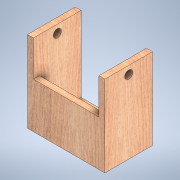
# Autodesk Inventor part: woodForkAssembly02
Saved by Autodesk Inventor 2022.2 (Build 262287000, 287)
## iProperties
Created: 2020-07-02
Part Number: woodForkAssembly02
Material: Wood (Birch)
Document SubType Name: Modeling
Designer: robst
Density: 0.55 g/cm^3
Appearance: Birch - Natural Polished
Mass: 1433.83 g
Surface Area: 3055.89 cm^2
Volume: 2606.97 cm^3
Author: robst
Autodesk Inventor part; units mm, degrees
ref_plane "YZ Plane" through (0, 0, 0) normal (1, 0, 0) x (0, 1, 0)
ref_plane "XZ Plane" through (0, 0, 0) normal (0, 1, 0) x (-1, 0, 0)
ref_plane "XY Plane" through (0, 0, 0) normal (0, 0, 1) x (1, 0, 0)
sketch "Sketch1" plane through (0, 0, 0) normal (0, 1, 0) x (-1, 0, 0)
  line L0 (123.825, 76.2) -> (-123.825, 76.2)
  line L1 (-123.825, 76.2) -> (-123.825, -76.2)
  line L2 (-123.825, -76.2) -> (123.825, -76.2)
  line L3 (123.825, -76.2) -> (123.825, 76.2)
  line L4 (123.825, 76.2) -> (-123.825, -76.2) construction
  line L5 (-123.825, 76.2) -> (123.825, -76.2) construction
  point P0 (0, 0)
  dimension "d0" = 247.65
  dimension "d1" = 152.4
  constraints: 12 end point, 2 midpoint, 2 parallel, 1 horizontal, 1 perpendicular
  measures "d0" distance of L0.start L0.end
  measures "d1" distance of L1.end L0.end
extrude "Extrusion1" add sketch "Sketch1" against normal blind 19.05
sketch "Sketch2" plane through (0, 0, 0) normal (0, 1, 0) x (1, 0, 0)
  line L0 (-123.825, -76.2) -> (-123.825, 76.2) projected
  line L1 (-123.825, 76.2) -> (-104.775, 76.2)
  line L2 (-104.775, 76.2) -> (-104.775, -76.2)
  line L3 (-104.775, -76.2) -> (-123.825, -76.2)
  line L4 (-123.825, -76.2) -> (-123.825, 76.2)
  line L5 (123.825, 76.2) -> (123.825, -76.2) projected
  line L6 (123.825, -76.2) -> (-123.825, -76.2) projected
  line L7 (123.825, 76.2) -> (104.775, 76.2)
  line L8 (104.775, 76.2) -> (104.775, -76.2)
  line L9 (104.775, -76.2) -> (123.825, -76.2)
  line L10 (123.825, -76.2) -> (123.825, 76.2)
  line L11 (-123.825, -76.2) -> (123.825, -76.2) projected
  point P0 (0, 0)
  dimension "d4" = 19.05
  constraints: 16 end point, 4 parallel, 2 collinear, 2 horizontal, 2 perpendicular, 1 point on line
  measures "d4" distance of L0.end L1.end
extrude "Extrusion2" add sketch "Sketch2" along normal blind 241.3
sketch "Sketch3" plane through (0, 0, 0) normal (0, 1, 0) x (1, 0, 0)
  line L0 (-123.825, -76.2) -> (-104.775, -76.2) projected
  line L1 (104.775, 76.2) -> (104.775, -76.2) projected
  line L2 (-104.775, -76.2) -> (104.775, -76.2)
  line L3 (104.775, -76.2) -> (104.775, -57.15)
  line L4 (104.775, -57.15) -> (-104.775, -57.15)
  line L5 (-104.775, -57.15) -> (-104.775, -76.2)
  point P0 (0, 0)
  dimension "d7" = 19.05
  constraints: 8 end point, 2 parallel, 1 horizontal, 1 perpendicular, 1 point on line
  measures "d7" distance of L4.end L0.end
extrude "Extrusion3" add sketch "Sketch3" along normal blind 127
sketch "Sketch5" plane through (123.825, -19.05, 76.2) normal (1, 0, 0) x (0, 0, -1)
  line L0 (152.4, 260.35) -> (0, 260.35) construction
  line L1 (76.2, 260.35) -> (76.2, 0) construction
  line L2 (0, 0) -> (152.4, 0) construction
  line L3 (19.05, 19.05) -> (152.4, 19.05) projected
  point P0 (76.2, 19.05)
  point P1 (76.2, 234.95)
  dimension "d23" = 215.9
  constraints: 2 end point, 2 midpoint, 1 point on line
  measures "d23" distance from line of point (76.2, 234.95) L3
hole "Hole1" at (123.825, 215.9, 0) direction (-1, 0, 0) diameter 25.908 end through all
equation "\"d0\" = interiorWidth + 2 * woodThickness"
equation "\"d1\" = partDepth"
equation "\"d2\" = woodThickness"
equation "\"d4\" = woodThickness"
equation "\"d5\" = totalHeight - woodThickness"
equation "\"d7\" = woodThickness"
equation "\"d8\" = supportBoardHeight"
equation "\"d23\" = holeCenter"
equation "\"d13\" = holeDiameter"
equation "\"interiorWidth\" = 209.55"
equation "\"woodThickness\" = 19.05"
equation "\"holeCenter\" = 215.9"
equation "\"supportBoardHeight\" = 127"
equation "\"holeDiameter\" = 25.908"
equation "\"partDepth\" = 152.4"
equation "\"totalHeight\" = 260.35"
body "Solid1"
